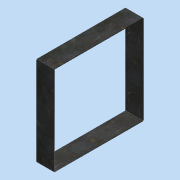
# Autodesk Inventor part: Aussengehäuse
Saved by Autodesk Inventor 2015 SP1 (Build 190203100, 203)
## iProperties
Created: 2015-04-14
Part Number: Aussengehäuse
Material: Stahl
Document SubType Name: Modeling
Designer: ElMatinho
Density: 7.85 g/cm^3
Appearance: Platte
Author: ElMatinho
Autodesk Inventor part; units mm, degrees
ref_plane "YZ Plane" through (0, 0, 0) normal (1, 0, 0) x (0, 1, 0)
ref_plane "XZ Plane" through (0, 0, 0) normal (0, 1, 0) x (-1, 0, 0)
ref_plane "XY Plane" through (0, 0, 0) normal (0, 0, 1) x (1, 0, 0)
sketch "Skizze1" plane through (0, 0, 0) normal (1, 0, 0) x (0, 1, 0)
  line L0 (0, -178.5) -> (0, 178.5) projected
  line L1 (-178.5, 0) -> (178.5, 0) projected
  line L2 (127.5, 127.5) -> (-127.5, 127.5)
  line L3 (-127.5, 127.5) -> (-127.5, -127.5)
  line L4 (-127.5, -127.5) -> (127.5, -127.5)
  line L5 (127.5, -127.5) -> (127.5, 127.5)
  point P0 (0, 0)
  dimension "d0" = 255
  dimension "d1" = 255
  constraints: 8 end point, 2 parallel, 1 horizontal, 1 perpendicular, 2 other
  measures "d0" distance of L4.end L2.start
  measures "d1" distance of L2.start L2.end
extrude "Extrusion1" add sketch "Skizze1" along normal mid plane 50
sketch "Skizze2" plane through (25, 0, 0) normal (1, 0, 0) x (0, 0, -1)
  line L0 (0, -178.5) -> (0, 178.5) projected
  line L1 (178.5, 0) -> (-178.5, 0) projected
  line L2 (-126, 126) -> (126, 126)
  line L3 (126, 126) -> (126, -126)
  line L4 (126, -126) -> (-126, -126)
  line L5 (-126, -126) -> (-126, 126)
  point P0 (0, 0)
  dimension "d4" = 252
  dimension "d5" = 252
  constraints: 8 end point, 2 parallel, 1 horizontal, 1 perpendicular, 2 other
  measures "d4" distance of L2.start L2.end
  measures "d5" distance of L4.end L2.start
extrude "Extrusion2" cut sketch "Skizze2" against normal blind 50
fillet "Rundung1" radius 2.5 4 edges at (0, 127.5, 127.5) (0, 127.5, -127.5) (0, -127.5, 127.5) (0, -127.5, -127.5)
fillet "Rundung2" radius 1 4 edges at (0, 126, 126) (0, 126, -126) (0, -126, -126) (0, -126, 126)
sketch "Skizze3" plane through (25, -126, 125) normal (0, 1, 0) x (1, 0, 0)
  circle A0 centre (-35, 51) radius 2
  circle A1 centre (-35, 199) radius 2
  line L0 (0, 0) -> (-50, 0) projected
  line L1 (-50, 0) -> (-50, 250) projected
  point P0 (-50, -1)
  dimension "d15" = 4
  dimension "d16" = 4
  dimension "d19" = 52
  dimension "d20" = 148
  dimension "d21" = 15
  dimension "d22" = 15
  constraints: 2 centre point
  measures "d15" diameter of A0
  measures "d16" diameter of A1
  measures "d19" vertical distance of point (-50, -1) A0.centre
  measures "d20" distance of A0.centre A1.centre
  measures "d21" distance from line of L1 A1.centre
  measures "d22" distance from line of L1 A0.centre
extrude "Extrusion3" add sketch "Skizze3" along normal blind 10
sketch "Skizze4" plane through (25, 126, -125) normal (0, -1, 0) x (1, 0, 0)
  circle A0 centre (-35, 51) radius 2
  circle A1 centre (-35, 199) radius 2
  line L0 (-50, 0) -> (-50, 250) projected
  point P0 (-25, 125)
  point P1 (-50, -1)
  dimension "d23" = 4
  dimension "d24" = 4
  dimension "d25" = 15
  dimension "d26" = 15
  dimension "d27" = 52
  dimension "d28" = 148
  constraints: 2 centre point
  measures "d23" diameter of A0
  measures "d24" diameter of A1
  measures "d25" distance from line of L0 A1.centre
  measures "d26" distance from line of L0 A0.centre
  measures "d27" vertical distance of point (-50, -1) A0.centre
  measures "d28" distance of A1.centre A0.centre
extrude "Extrusion4" add sketch "Skizze4" along normal blind 10
